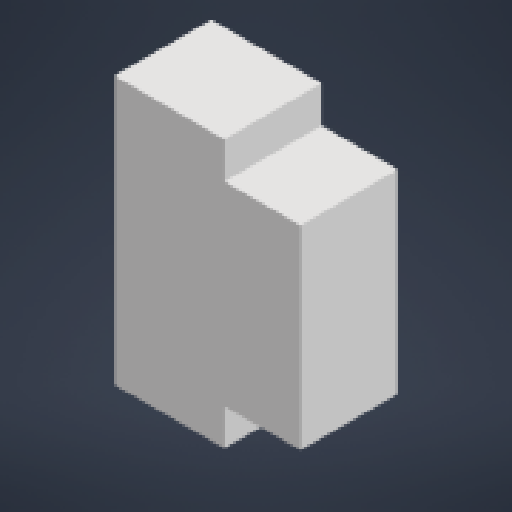
# Autodesk Inventor part: ESPLED
Saved by Autodesk Inventor 2023 (Build 270158000, 158)
## iProperties
Created: 2022-10-27
Part Number: ESPLED
Material: Generic
Document SubType Name: Modeling
Designer: jevan
Density: 1 g/cm^3
Appearance: Default
Author: jevan
Autodesk Inventor part; units mm, degrees
ref_plane "YZ Plane" through (0, 0, 0) normal (1, 0, 0) x (0, 1, 0)
ref_plane "XZ Plane" through (0, 0, 0) normal (0, 1, 0) x (-1, 0, 0)
ref_plane "XY Plane" through (0, 0, 0) normal (0, 0, 1) x (1, 0, 0)
sketch "Sketch1" plane through (0, 0, 0) normal (0, 0, 1) x (1, 0, 0)
  line L0 (0, 0) -> (0.68, 0)
  line L1 (0.68, 0) -> (0.68, -1.65)
  line L2 (0.68, -1.65) -> (0, -1.65)
  line L3 (0, -1.65) -> (0, 0)
  line L4 (0.68, -0.825) -> (1.15, -0.825)
  line L5 (1.15, -0.825) -> (1.15, -1.425)
  line L6 (1.15, -1.425) -> (0.68, -1.425)
  line L7 (1.15, -0.825) -> (1.15, -0.225)
  line L8 (1.15, -0.225) -> (0.68, -0.225)
  dimension "d0" = 0.68
  dimension "d1" = 1.65
  dimension "d2" = 0.47
  dimension "d3" = 0.6
  dimension "d4" = 0.6
  constraints: 18 end point, 4 perpendicular, 3 point on line, 2 horizontal, 2 parallel, 1 midpoint
  measures "d0" distance of L1.end L2.end
  measures "d1" distance of L0.end L1.end
  measures "d2" distance of L4.start L4.end
  measures "d3" distance of L4.end L5.end
  measures "d4" distance of L4.end L7.end
extrude "Extrusion1" add sketch "Sketch1" along normal blind 0.6
body "Solid1"
